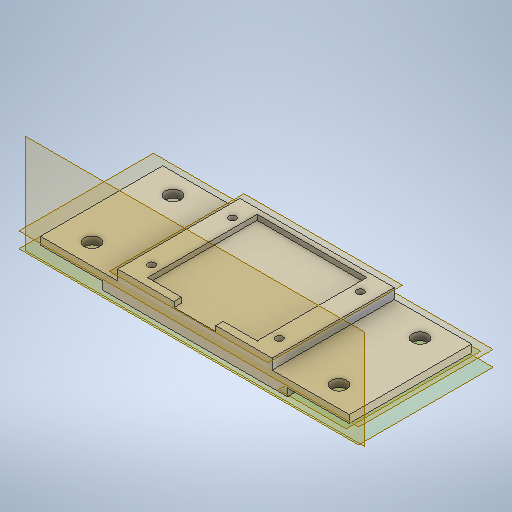
# Autodesk Inventor part: motor_mount1
Saved by Autodesk Inventor 2025.2 (Build 292293000, 293)
## iProperties
Created: 2024-12-22
Part Number: motor_mount1
Material: 一般
Document SubType Name: Modeling
Designer: mahhy
Density: 1 g/cm^3
Appearance: 既定
Author: mahhy
## iProperties of the stored document motor_mount1_3D プリント.ipt
Created: 2024-12-22
Part Number: motor_mount1_3D プリント
Material: 一般
Document SubType Name: Modeling
Designer: mahhy
Density: 1 g/cm^3
Appearance: 既定
Author: mahhy
Autodesk Inventor part; units mm, degrees
ref_plane "YZ Plane" through (0, 0, 0) normal (1, 0, 0) x (0, 1, 0)
ref_plane "XZ Plane" through (0, 0, 0) normal (0, 1, 0) x (-1, 0, 0)
ref_plane "XY Plane" through (0, 0, 0) normal (0, 0, 1) x (1, 0, 0)
sketch "スケッチ1" plane through (0, 0, 0) normal (0, 1, 0) x (-1, 0, 0)
  line L0 (0, 0) -> (-120, 0)
  line L1 (-120, 0) -> (-120, -47.5)
  line L2 (-120, -47.5) -> (0, -47.5)
  line L3 (0, -47.5) -> (0, 0)
  dimension "d0" = 120
  dimension "d1" = 47.5
  constraints: 8 end point, 2 parallel, 1 horizontal, 1 perpendicular
  measures "d0" distance of L2.end L1.end
  measures "d1" distance of L1.end L0.end
extrude "押し出し1" add sketch "スケッチ1" along normal blind 6
ref_plane "作業平面1" through (0, 0, 0) normal (0, 0, 1) x (1, 0, 0)
ref_plane "作業平面2" through (0, 6, 0) normal (0, 1, 0) x (1, 0, 0)
sketch "スケッチ3" plane through (0, 6, 0) normal (0, 1, 0) x (1, 0, 0)
  line L0 (120, 47.5) -> (0, 47.5) projected
  line L1 (0, 0) -> (120, 0) projected
  line L2 (30, 47.5) -> (90, 47.5)
  line L3 (90, 47.5) -> (90, 0)
  line L4 (90, 0) -> (30, 0)
  line L5 (30, 0) -> (30, 47.5)
  point P0 (30, 0)
  point P1 (60, 47.5)
  point P2 (60, 47.5)
  point P3 (60, 47.5)
  dimension "d9" = 60
  dimension "d50" = 0
  constraints: 8 end point, 3 midpoint, 2 parallel, 2 point on line, 1 horizontal, 1 perpendicular
  measures "d9" distance of L3.end L4.end
  measures "d50" distance of point (60, 47.5) point (60, 47.5)
extrude "押し出し3" add sketch "スケッチ3" along normal blind 4
ref_plane "作業平面3" through (0, 10, 0) normal (0, 1, 0) x (1, 0, 0)
sketch "スケッチ4" plane through (0, 10, 0) normal (0, 1, 0) x (1, 0, 0)
  line L0 (38.7, 45.5) -> (81.3, 45.5)
  line L1 (81.3, 45.5) -> (81.3, 2.9)
  line L2 (81.3, 2.9) -> (38.7, 2.9)
  line L3 (38.7, 2.9) -> (38.7, 45.5)
  line L4 (90, 47.5) -> (30, 47.5) projected
  line L5 (90, 0) -> (90, 47.5) projected
  point P0 (0, 0)
  point P1 (90, 23.75)
  point P2 (60, 47.5)
  dimension "d14" = 42.6
  dimension "d15" = 42.6
  constraints: 8 end point, 2 midpoint, 2 parallel, 1 horizontal, 1 perpendicular
  measures "d14" distance of L1.end L2.end
  measures "d15" distance of L0.end L1.end
extrude "押し出し4" cut sketch "スケッチ4" against normal blind 2
sketch "スケッチ5" plane through (120, 0, 0) normal (0, 0, 1) x (1, 0, 0)
  line L0 (-30, 10) -> (-90, 10) projected
  line L1 (-38.7, 8) -> (-81.3, 8) projected
  line L2 (-68.1, 10) -> (-51.9, 10)
  line L3 (-51.9, 10) -> (-51.9, 8)
  line L4 (-51.9, 8) -> (-68.1, 8)
  line L5 (-68.1, 8) -> (-68.1, 10)
  point P0 (-120, 0)
  dimension "d20" = 16.2
  constraints: 8 end point, 2 parallel, 2 point on line, 1 horizontal, 1 perpendicular
  measures "d20" distance of L3.end L4.end
extrude "押し出し5" cut sketch "スケッチ5" against normal blind 3
sketch "スケッチ6" plane through (0, 10, 0) normal (0, 1, 0) x (1, 0, 0)
  line L0 (90, 47.5) -> (30, 47.5) projected
  line L1 (144, 0) -> (-24, 0) projected
  line L2 (30, 47.5) -> (30, 0) projected
  line L3 (90, 0) -> (90, 47.5) projected
  point P0 (0, 0)
  point P1 (35.2, 39.5)
  point P2 (35.2, 8)
  point P3 (84.8, 8)
  point P4 (84.8, 39.5)
  dimension "d27" = 8
  dimension "d28" = 8
  dimension "d29" = 8
  dimension "d30" = 8
  dimension "d31" = 5.2
  dimension "d32" = 5.2
  dimension "d33" = 5.2
  dimension "d34" = 5.2
  dimension "d49" = 49.6
  measures "d27" distance from line of L0 point (35.2, 39.5)
  measures "d28" distance from line of L0 point (84.8, 39.5)
  measures "d29" distance from line of L1 point (84.8, 8)
  measures "d30" distance from line of L1 point (35.2, 8)
  measures "d31" distance from line of L2 point (35.2, 39.5)
  measures "d32" distance from line of L2 point (35.2, 8)
  measures "d33" distance from line of L3 point (84.8, 39.5)
  measures "d34" distance from line of L3 point (84.8, 8)
  measures "d49" distance of point (84.8, 39.5) point (35.2, 39.5)
hole "穴1" at (35.2, 10, -39.5) at (35.2, 10, -8) at (84.8, 10, -8) at (84.8, 10, -39.5) direction (0, -1, 0) diameter 2.8 end through all
sketch "スケッチ7" plane through (0, 0, 0) normal (0, -1, 0) x (1, 0, 0)
  circle A0 centre (35.2, -8) radius 1.4 projected
  circle A1 centre (35.2, -8) radius 3.5
  circle A2 centre (84.8, -8) radius 1.4 projected
  circle A3 centre (84.8, -8) radius 3.5
  circle A4 centre (84.8, -39.5) radius 1.4 projected
  circle A5 centre (84.8, -39.5) radius 3.5
  circle A6 centre (35.2, -39.5) radius 1.4 projected
  circle A7 centre (35.2, -39.5) radius 3.5
  point P0 (0, 0)
  dimension "d42" = 7
  dimension "d43" = 7
  dimension "d44" = 7
  dimension "d45" = 7
  constraints: 4 centre point, 4 coincident
  measures "d42" diameter of A1
  measures "d43" diameter of A3
  measures "d44" diameter of A5
  measures "d45" diameter of A7
extrude "押し出し6" cut sketch "スケッチ7" against normal blind 4 contours A0 | A1 | A3 | A4 | A5 | A6 | A7
ref_plane "作業平面4" through (0, 0, 0) normal (0, -1, 0) x (1, 0, 0)
sketch "スケッチ8" plane through (0, 0, 0) normal (0, -1, 0) x (1, 0, 0)
  line L0 (0, 0) -> (24, 0)
  line L1 (24, 0) -> (24, -47.5)
  line L2 (24, -47.5) -> (0, -47.5)
  line L3 (0, -47.5) -> (0, 0)
  line L4 (120, 0) -> (120, -47.5) projected
  line L5 (120, 0) -> (96, 0)
  line L6 (96, 0) -> (96, -47.5)
  line L7 (96, -47.5) -> (120, -47.5)
  line L8 (120, -47.5) -> (120, 0)
  dimension "d53" = 24
  dimension "d54" = 47.5
  dimension "d55" = 24
  dimension "d56" = 47.5
  constraints: 16 end point, 4 parallel, 2 horizontal, 2 perpendicular
  measures "d53" distance of L1.end L2.end
  measures "d54" distance of L0.end L1.end
  measures "d55" distance of L7.end L6.end
  measures "d56" distance of L6.end L5.end
extrude "押し出し7" cut sketch "スケッチ8" against normal blind 3
ref_plane "作業平面5" through (0, 3, 0) normal (0, -1, 0) x (1, 0, 0)
sketch "スケッチ9" plane through (0, 3, 0) normal (0, -1, 0) x (1, 0, 0)
  line L0 (0, -47.5) -> (0, 0) projected
  line L1 (0, 0) -> (24, 0) projected
  line L2 (24, -47.5) -> (0, -47.5) projected
  line L3 (120, 0) -> (120, -47.5) projected
  line L4 (96, 0) -> (120, 0) projected
  line L5 (120, -47.5) -> (96, -47.5) projected
  point P0 (12, -8)
  point P1 (12, -39.5)
  point P2 (108, -8)
  point P3 (108, -39.5)
  point P4 (12, 0)
  dimension "d60" = 12
  dimension "d61" = 8
  dimension "d62" = 8
  dimension "d63" = 12
  dimension "d64" = 12
  dimension "d65" = 12
  dimension "d66" = 8
  dimension "d67" = 8
  constraints: 1 midpoint
  measures "d60" distance from line of L0 point (12, -8)
  measures "d61" distance of point (12, 0) point (12, -8)
  measures "d62" distance from line of L2 point (12, -39.5)
  measures "d63" distance from line of L0 point (12, -39.5)
  measures "d64" distance from line of L3 point (108, -39.5)
  measures "d65" distance from line of L3 point (108, -8)
  measures "d66" distance from line of L4 point (108, -8)
  measures "d67" distance from line of L5 point (108, -39.5)
hole "穴2" at (12, 3, -8) at (12, 3, -39.5) at (108, 3, -8) at (108, 3, -39.5) direction (0, 1, 0) diameter 6 end through all
